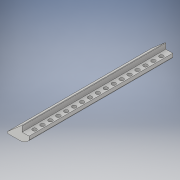
# Autodesk Inventor part: Ramp 2
Saved by Autodesk Inventor 2019 (Build 230136000, 136)
## iProperties
Created: 2019-01-25
Part Number: Ramp 2
Material: Generic
Document SubType Name: Modeling
Designer: Ashley
Density: 1 g/cm^3
Appearance: Default
Author: Ashley
Autodesk Inventor part; units mm, degrees
ref_plane "YZ Plane" through (0, 0, 0) normal (1, 0, 0) x (0, 1, 0)
ref_plane "XZ Plane" through (0, 0, 0) normal (0, 1, 0) x (-1, 0, 0)
ref_plane "XY Plane" through (0, 0, 0) normal (0, 0, 1) x (1, 0, 0)
sketch "Sketch1" plane through (0, 0, 0) normal (0, 0, 1) x (1, 0, 0)
  line L0 (11, 16) -> (11, 0) construction
  line L1 (11, 0) -> (-11, 0) construction
  line L2 (-11, 0) -> (-11, 1.5)
  line L3 (0, 16) -> (0, 0) construction
  line L4 (4, 14.5) -> (-11, 1.5)
  line L5 (4, 14.5) -> (4, 8.5)
  line L6 (4, 14.5) -> (10, 14.5) construction
  line L7 (4, 8.5) -> (11, 8.5)
  line L8 (11, 4.5) -> (5.3133, 0)
  line L9 (11, 4.5) -> (11, 8.5)
  line L10 (-11, 0) -> (5.3133, 0)
  dimension "d3" = 1.5
  dimension "d10" = 7
  dimension "d12" = 22
  dimension "d13" = 6
  dimension "d14" = 130.914
  dimension "d15" = 90
  dimension "d16" = 49.086
  dimension "d17" = 90
  dimension "d18" = 90
  dimension "d19" = 90
  dimension "d20" = 141.645
  dimension "d21" = 128.355
  dimension "d22" = 4
  constraints: 22 end point, 3 point on line, 2 collinear, 2 midpoint, 2 perpendicular, 1 horizontal, 1 parallel, 1 vertical
  measures "d3" distance of L2.end L1.end
  measures "d10" distance of L5.end L7.end
  measures "d12" distance of L0.end L1.end
  measures "d13" distance of L4.start L5.end
  measures "d14" angle of L2 L4
  measures "d15" angle of L5 L7
  measures "d16" angle of L4 L5
  measures "d17" angle of L0 L7
  measures "d18" angle of L2 L1
  measures "d19" angle of L1 L0
  measures "d20" angle of L10 L8
  measures "d21" angle of L8 L9
  measures "d22" distance of L8.start L7.end
extrude "Extrusion1" add sketch "Sketch1" along normal blind 145
fillet "Fillet1" radius 1 1 edges at (-11, 0, 72.5)
fillet "Fillet2" radius 1 1 edges at (-11, 1.5, 72.5)
fillet "Fillet3" radius 10 1 edges at (5.3133, 0, 72.5)
fillet "Fillet5" radius 0.3 1 edges at (4, 14.5, 72.5)
sketch "Sketch2" plane through (4, 8.5, 145) normal (0, 1, 0) x (1, 0, 0)
  line L0 (6.6447, 145) -> (6.6447, 0) construction
  line L1 (0, 145) -> (0, 0) construction
  circle A0 centre (4, 8.5) radius 2
  circle A1 centre (4, 16.5) radius 2
  circle A2 centre (4, 24.5) radius 2
  circle A3 centre (4, 32.5) radius 2
  circle A4 centre (4, 40.5) radius 2
  circle A5 centre (4, 48.5) radius 2
  circle A6 centre (4, 56.5) radius 2
  circle A7 centre (4, 64.5) radius 2
  circle A8 centre (4, 72.5) radius 2
  circle A9 centre (4, 80.5) radius 2
  circle A10 centre (4, 88.5) radius 2
  circle A11 centre (4, 96.5) radius 2
  circle A12 centre (4, 104.5) radius 2
  circle A13 centre (4, 112.5) radius 2
  circle A14 centre (4, 120.5) radius 2
  circle A15 centre (4, 128.5) radius 2
  circle A16 centre (4, 136.5) radius 2
  line L2 (4, 8.5) -> (4, 16.5) construction
  line L3 (4, 16.5) -> (4, 24.5) construction
  line L4 (4, 24.5) -> (4, 32.5) construction
  line L5 (4, 32.5) -> (4, 40.5) construction
  line L6 (4, 40.5) -> (4, 48.5) construction
  line L7 (4, 48.5) -> (4, 56.5) construction
  line L8 (4, 56.5) -> (4, 64.5) construction
  line L9 (4, 64.5) -> (4, 72.5) construction
  line L10 (4, 72.5) -> (4, 80.5) construction
  line L11 (4, 80.5) -> (4, 88.5) construction
  line L12 (4, 88.5) -> (4, 96.5) construction
  line L13 (4, 96.5) -> (4, 104.5) construction
  line L14 (4, 104.5) -> (4, 112.5) construction
  line L15 (4, 112.5) -> (4, 120.5) construction
  line L16 (4, 120.5) -> (4, 128.5) construction
  line L17 (4, 128.5) -> (4, 136.5) construction
  line L18 (4, 136.5) -> (4, 144.5) construction
  line L19 (4, 72.5) -> (-64.0326, 72.5) construction
  point P0 (6.6447, 72.5)
  dimension "d32" = 4
  constraints: 38 end point, 30 collinear, 17 centre point, 2 parallel, 1 horizontal, 1 midpoint, 1 point on line
  measures "d32" distance from line of L1 L9.end
extrude "Extrusion2" cut sketch "Sketch2" against normal through all
fillet "Fillet6" radius 1 1 edges at (11, 4.5, 72.5)
body "Solid1"
